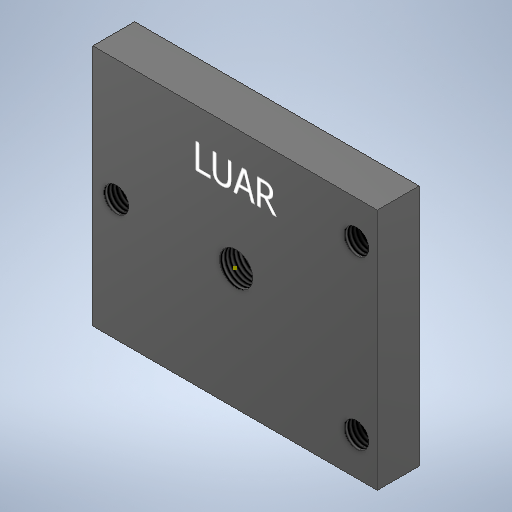
# Autodesk Inventor part: Part2
Saved by Autodesk Inventor 2025.1 (Build 291241000, 241)
## iProperties
Created: 2024-09-22
Part Number: Part2
Material: ABS Plastic
Document SubType Name: Modeling
Designer: JuhenFW
Density: 1.06 g/cm^3
Appearance: Smooth - White
Author: JuhenFW
Autodesk Inventor part; units mm, degrees
ref_plane "YZ Plane" through (0, 0, 0) normal (1, 0, 0) x (0, 1, 0)
ref_plane "XZ Plane" through (0, 0, 0) normal (0, 1, 0) x (-1, 0, 0)
ref_plane "XY Plane" through (0, 0, 0) normal (0, 0, 1) x (1, 0, 0)
sketch "Sketch1" plane through (0, 0, 0) normal (0, 0, 1) x (1, 0, 0)
  point P0 (0, 0)
sketch "Sketch2" plane through (0, 0, 0) normal (0, 0, 1) x (1, 0, 0)
  line L0 (-17, -14.5) -> (17, -14.5)
  line L1 (17, -14.5) -> (17, 14.5)
  line L2 (17, 14.5) -> (-17, 14.5)
  line L3 (-17, 14.5) -> (-17, -14.5)
  circle A0 centre (14.5, 10) radius 1.5
  circle A1 centre (14.5, -10) radius 1.5
  circle A2 centre (-14.2, 0) radius 1.5
  point P0 (0, 0)
  dimension "d0" = 34
  dimension "d1" = 29
  dimension "d2" = 3
  dimension "d3" = 3
  dimension "d4" = 3
  dimension "d5" = 20
  dimension "d6" = 2.5
  dimension "d7" = 14.5
  dimension "d8" = 28.7
  constraints: 8 end point, 3 centre point, 2 parallel, 1 horizontal, 1 perpendicular, 1 vertical alignment
  measures "d0" distance of L2.end L1.end
  measures "d1" distance between parallel lines of L0 L2
  measures "d2" diameter of A0
  measures "d3" diameter of A1
  measures "d4" diameter of A2
  measures "d5" distance of A1.centre A0.centre
  measures "d6" distance from line of L1 A1.centre
  measures "d7" distance from line of L2 A2.centre
  measures "d8" horizontal distance of A0.centre A2.centre
extrude "Extrusion1" add sketch "Sketch2" along normal blind 5
thread "Thread1" size "M3x0.5" class "6H" standard "ANSI Metric M Profile" length 5
thread "Thread2" size "M3x0.5" class "6H" standard "ANSI Metric M Profile" length 5
thread "Thread3" size "M3x0.5" class "6H" standard "ANSI Metric M Profile" length 5
sketch "Sketch3" plane through (0, 0, 5) normal (0, 0, 1) x (1, 0, 0)
  line L0 (-7.3481, 13.6395) -> (7.272, 13.6395) construction
  line L1 (7.272, 13.6395) -> (7.272, 4.876) construction
  line L2 (7.272, 4.876) -> (-7.3481, 4.876) construction
  line L3 (-7.3481, 4.876) -> (-7.3481, 13.6395) construction
  point P0 (0, 0)
  dimension "d0" = 34
  dimension "d1" = 29
  dimension "d2" = 3
  dimension "d3" = 3
  dimension "d4" = 3
  dimension "d5" = 20
  dimension "d6" = 2.5
  dimension "d7" = 14.5
  dimension "d8" = 28.7
  constraints: 2 other
sketch "Sketch4" plane through (0, 0, 5) normal (0, 0, 1) x (1, 0, 0)
  circle A0 centre (0.125, 0) radius 2
  circle A1 centre (14.5, 10) radius 1.5 projected
  circle A2 centre (-14.2, 0) radius 1.5 projected
  dimension "d18" = 4
  dimension "d21" = 14.375
  constraints: 1 centre point, 1 coincident
  measures "d18" diameter of A0
  measures "d21" horizontal distance of A1.centre point (0.125, 0)
extrude "Extrusion2" cut sketch "Sketch4" against normal blind 5 contours A0
thread "Thread4" size "M4x0.5" class "6H" standard "ANSI Metric M Profile" length 5
body "Solid1"
